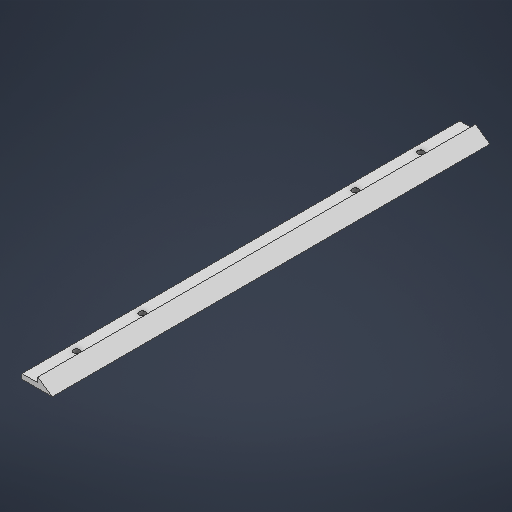
# Autodesk Inventor part: plug
Saved by Autodesk Inventor 2026.2 (Build 302298010, 298A)
## iProperties
Created: 2026-09-28
Part Number: plug
Material: Generic
Document SubType Name: Modeling
Designer: karol
Density: 1 g/cm^3
Appearance: Default
Author: karol
Autodesk Inventor part; units mm, degrees
ref_plane "YZ Plane" through (0, 0, 0) normal (1, 0, 0) x (0, 1, 0)
ref_plane "XZ Plane" through (0, 0, 0) normal (0, 1, 0) x (-1, 0, 0)
ref_plane "XY Plane" through (0, 0, 0) normal (0, 0, 1) x (1, 0, 0)
sketch "Sketch1" plane through (0, 0, 0) normal (0, 0, 1) x (1, 0, 0)
  line L0 (0, 0) -> (12.5, 0)
  line L1 (0, 0) -> (0, 2)
  line L2 (0, 2) -> (6.5, 2)
  line L3 (6.5, 2) -> (6.5, 4)
  line L4 (6.5, 4) -> (12.5, 0)
  dimension "d0" = 12.5
  dimension "d1" = 2
  dimension "d2" = 6.5
  dimension "d3" = 2
  constraints: 10 end point, 2 perpendicular, 1 horizontal, 1 vertical
  measures "d0" distance of L0.start L0.end
  measures "d1" distance of L0.start L1.end
  measures "d2" distance of L1.end L2.end
  measures "d3" distance of L2.end L3.end
extrude "Extrusion1" add sketch "Sketch1" along normal blind 180
sketch "Sketch2" plane through (0, 2, 0) normal (0, 1, 0) x (1, 0, 0)
  circle A0 centre (3.25, -160.8) radius 1.25
  circle A1 centre (3.25, -133.8) radius 1.25
  circle A2 centre (3.25, -46.2) radius 1.25
  circle A3 centre (3.25, -19.2) radius 1.25
  line L0 (6.5, 0) -> (0, 0) projected
  line L1 (6.5, -180) -> (0, -180) projected
  line L2 (0, 0) -> (0, -180) projected
  point P0 (3.25, -180)
  dimension "d6" = 2.5
  dimension "d7" = 2.5
  dimension "d8" = 2.5
  dimension "d9" = 2.5
  dimension "d10" = 19.2
  dimension "d11" = 46.2
  dimension "d12" = 19.2
  dimension "d13" = 3.25
  dimension "d14" = 46.2
  dimension "d15" = 3.25
  dimension "d16" = 3.25
  dimension "d17" = 3.25
  constraints: 4 centre point, 1 midpoint
  measures "d6" diameter of A0
  measures "d7" diameter of A1
  measures "d8" diameter of A2
  measures "d9" diameter of A3
  measures "d10" distance from line of L0 A3.centre
  measures "d11" distance from line of L0 A2.centre
  measures "d12" distance of point (3.25, -180) A0.centre
  measures "d13" distance from line of L2 A0.centre
  measures "d14" distance from line of L1 A1.centre
  measures "d15" distance from line of L2 A1.centre
  measures "d16" distance from line of L2 A2.centre
  measures "d17" distance from line of L2 A3.centre
hole "Hole1" at (3.25, 2, 160.8) at (3.25, 2, 133.8) at (3.25, 2, 46.2) at (3.25, 2, 19.2) direction (0, -1, 0) diameter 2.459 depth 2 countersink diameter 2.5 countersink angle 90 thread size "M3x0.5" class "6H" standard "ANSI Metric M Profile"
body "Solid1"
